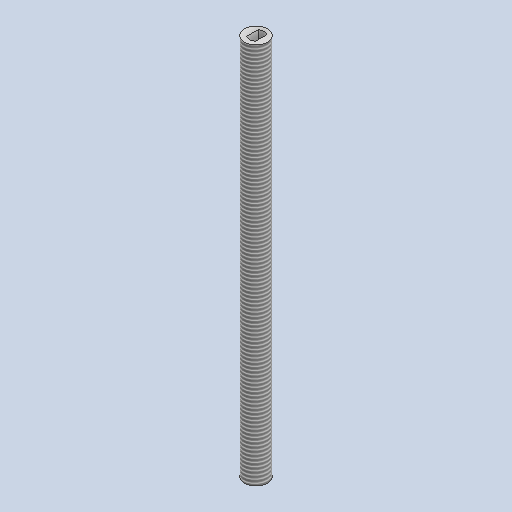
# Autodesk Inventor part: leadscrewaxle
Saved by Autodesk Inventor 2025.4 (Build 294407000, 407)
## iProperties
Created: 2026-03-22
Part Number: leadscrewaxle
Material: Generic
Document SubType Name: Modeling
Designer: hp
Density: 1 g/cm^3
Appearance: Default
Author: hp
Autodesk Inventor part; units mm, degrees
ref_plane "YZ Plane" through (0, 0, 0) normal (1, 0, 0) x (0, 1, 0)
ref_plane "XZ Plane" through (0, 0, 0) normal (0, 1, 0) x (-1, 0, 0)
ref_plane "XY Plane" through (0, 0, 0) normal (0, 0, 1) x (1, 0, 0)
sketch "Sketch1" plane through (0, 0, 0) normal (0, 1, 0) x (-1, 0, 0)
  circle A0 centre (0, 0) radius 4
  arc A1 (1.3559, 1.8559) -> (-1.6441, 1.8559) centre (-0.1441, -0.1441) ccw
  arc A2 (-1.6441, -2.1441) -> (1.3559, -2.1441) centre (-0.1441, -0.1441) ccw
  line L0 (1.3559, 1.7344) -> (1.3559, -2.0227)
  line L1 (-1.6441, -2.0227) -> (-1.6441, 1.7344)
  line L2 (-1.6441, 1.7344) -> (-1.6441, 1.8559)
  line L3 (-1.6441, -2.1441) -> (-1.6441, -2.0227)
  line L4 (1.3559, -2.0227) -> (1.3559, -2.1441)
  line L5 (1.3559, 1.8559) -> (1.3559, 1.7344)
  dimension "d0" = 8
  constraints: 12 end point, 4 point on circle, 3 centre point, 1 coincident
  measures "d0" diameter of A0
extrude "Extrusion1" add sketch "Sketch1" against normal blind 132
thread "Thread1" size "M8x1.25" class "6g" standard "ANSI Metric M Profile" full length
body "Solid1"
